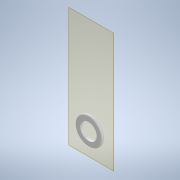
# Autodesk Inventor part: podkl
Saved by Autodesk Inventor 2021 (Build 250183000, 183)
## iProperties
Created: 2021-06-22
Part Number: podkl
Material: Stal, galwanizowana
Document SubType Name: Modeling
Designer: Wojciech Wołczek
Density: 7.85 g/cm^3
Appearance: Galwanizowana
Author: Wojciech Wołczek
Autodesk Inventor part; units mm, degrees
ref_plane "YZ Plane" through (0, 0, 0) normal (1, 0, 0) x (0, 1, 0)
ref_plane "XZ Plane" through (0, 0, 0) normal (0, 1, 0) x (-1, 0, 0)
ref_plane "XY Plane" through (0, 0, 0) normal (0, 0, 1) x (1, 0, 0)
ref_plane "Płaszczyzna konstrukcyjna1" through (0, 0, 0) normal (0, 0, 1) x (1, 0, 0)
sketch "Szkic1" plane through (0, 0, 0) normal (0, 0, 1) x (1, 0, 0)
  circle A0 centre (-0.0564, -13) radius 3 projected
  circle A1 centre (-0.0564, -13) radius 3
  circle A2 centre (-0.0564, -13) radius 10
  point P0 (0, 0)
  dimension "d0" = 6
  dimension "d1" = 20
  constraints: 2 centre point, 2 coincident
  measures "d0" diameter of A1
  measures "d1" diameter of A2
extrude "Wyciągnięcie proste1" add sketch "Szkic1" along normal blind 1
full round fillet "Zaokrąglenie1" first side at (7.4844, -14.037, 1) centre faces at (9.9112, -13.8047, 0.6667) second side at (7.4844, -14.037, 0)
